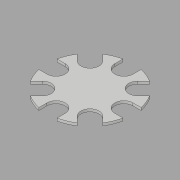
# Autodesk Inventor part: turntable
Saved by Autodesk Inventor 2017 (Build 210142000, 142)
## iProperties
Created: 2019-05-09
Part Number: turntable
Material: Generic
Document SubType Name: Modeling
Designer: Joe Sedutto
Density: 1 g/cm^3
Appearance: Default
Author: Joe Sedutto
Autodesk Inventor part; units mm, degrees
ref_plane "YZ Plane" through (0, 0, 0) normal (1, 0, 0) x (0, 1, 0)
ref_plane "XZ Plane" through (0, 0, 0) normal (0, 1, 0) x (-1, 0, 0)
ref_plane "XY Plane" through (0, 0, 0) normal (0, 0, 1) x (1, 0, 0)
sketch "Sketch1" plane through (0, 0, 0) normal (0, 1, 0) x (-1, 0, 0)
  circle A0 centre (0, 0) radius 34.925
  line L0 (0, 0) -> (0, -130.175) construction
  circle A1 centre (-92.0476, -38.1274) radius 34.925
  circle A2 centre (-130.175, -130.175) radius 34.925
  circle A3 centre (-92.0476, -222.2226) radius 34.925
  circle A4 centre (0, -260.35) radius 34.925
  circle A5 centre (92.0476, -222.2226) radius 34.925
  circle A6 centre (130.175, -130.175) radius 34.925
  circle A7 centre (92.0476, -38.1274) radius 34.925
  circle A8 centre (0, -130.175) radius 165.1
  dimension "d0" = 69.85
  dimension "d4" = 360
  dimension "d14" = 330.2
  constraints: 9 centre point, 2 coincident, 2 end point, 1 tangent, 1 vertical, 17 other
  measures "d0" diameter of A0
  measures "d14" diameter of A8
extrude "Extrusion1" add sketch "Sketch1" along normal blind 10
sketch "Sketch2" plane through (92.0476, 10, -38.1274) normal (0, 1, 0) x (1, 0, 0)
  arc A0 (-126.9726, -38.1274) -> (-57.1226, -38.1274) centre (-92.0476, -38.1274) ccw
  arc A1 (-126.9726, -69.3161) -> (-57.1226, -69.3161) centre (-92.0476, 92.0476) ccw
  line L0 (-57.1226, -38.1274) -> (-57.1226, -69.3161)
  line L1 (-126.9726, -38.1274) -> (-126.9726, -69.3161)
  circle A2 centre (-92.0476, -38.1274) radius 34.925 projected
  arc A3 (73.0524, 92.0476) -> (24.6957, 208.791) centre (-92.0476, 92.0476) ccw projected
  arc A4 (-24.6957, -24.6957) -> (24.6957, 24.6957) centre (0, 0) ccw
  arc A5 (-2.6419, -46.7495) -> (46.7495, 2.6419) centre (-92.0476, 92.0476) ccw
  line L2 (24.6957, 24.6957) -> (46.7495, 2.6419)
  line L3 (-24.6957, -24.6957) -> (-2.6419, -46.7495)
  arc A6 (38.1274, 57.1226) -> (38.1274, 126.9726) centre (38.1274, 92.0476) ccw
  arc A7 (69.3161, 57.1226) -> (69.3161, 126.9726) centre (-92.0476, 92.0476) ccw
  line L4 (38.1274, 126.9726) -> (69.3161, 126.9726)
  line L5 (38.1274, 57.1226) -> (69.3161, 57.1226)
  arc A8 (24.6957, 159.3995) -> (-24.6957, 208.791) centre (0, 184.0953) ccw
  arc A9 (46.7495, 181.4533) -> (-2.6419, 230.8447) centre (-92.0476, 92.0476) ccw
  line L6 (-24.6957, 208.791) -> (-2.6419, 230.8447)
  line L7 (24.6957, 159.3995) -> (46.7495, 181.4533)
  arc A10 (-57.1226, 222.2226) -> (-126.9726, 222.2226) centre (-92.0476, 222.2226) ccw
  arc A11 (-57.1226, 253.4114) -> (-126.9726, 253.4114) centre (-92.0476, 92.0476) ccw
  line L8 (-126.9726, 222.2226) -> (-126.9726, 253.4114)
  line L9 (-57.1226, 222.2226) -> (-57.1226, 253.4114)
  arc A12 (-159.3995, 208.791) -> (-208.791, 159.3995) centre (-184.0953, 184.0953) ccw
  arc A13 (-181.4533, 230.8447) -> (-230.8447, 181.4533) centre (-92.0476, 92.0476) ccw
  line L10 (-208.791, 159.3995) -> (-230.8447, 181.4533)
  line L11 (-159.3995, 208.791) -> (-181.4533, 230.8447)
  arc A14 (-222.2226, 126.9726) -> (-222.2226, 57.1226) centre (-222.2226, 92.0476) ccw
  arc A15 (-253.4114, 126.9726) -> (-253.4114, 57.1226) centre (-92.0476, 92.0476) ccw
  line L12 (-222.2226, 57.1226) -> (-253.4114, 57.1226)
  line L13 (-222.2226, 126.9726) -> (-253.4114, 126.9726)
  arc A16 (-208.791, 24.6957) -> (-159.3995, -24.6957) centre (-184.0953, 0) ccw
  arc A17 (-230.8447, 2.6419) -> (-181.4533, -46.7495) centre (-92.0476, 92.0476) ccw
  line L14 (-159.3995, -24.6957) -> (-181.4533, -46.7495)
  line L15 (-208.791, 24.6957) -> (-230.8447, 2.6419)
  point P0 (-92.0476, -73.0524)
  point P1 (-92.0476, -73.0524)
  point P2 (24.6957, -24.6957)
  point P3 (73.0524, 92.0476)
  point P4 (24.6957, 208.791)
  point P5 (-92.0476, 257.1476)
  point P6 (-208.791, 208.791)
  point P7 (-257.1476, 92.0476)
  point P8 (-208.791, -24.6957)
  dimension "d10" = 360
  constraints: 42 point on circle, 32 end point, 16 centre point, 4 coincident, 2 tangent, 1 parallel, 1 vertical, 87 other
extrude "Extrusion2" cut sketch "Sketch2" against normal blind 10 contours A0 A1 L1 | A0 L0 A1 | A6 L4 A3 | A7 L5 A6 | L7 A8 A3 | A8 L6 A9 | A4 L2 A5 | A4 A5 L3 | A10 L8 A11 | A10 A11 L9 | A12 L10 A13 | A12 A13 L11 | A14 L12 A15 | A14 A15 L13 | A16 L14 A17 | A16 A17 L15
body "Solid1"
